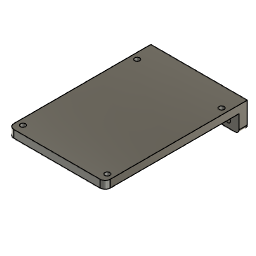
monitor holder v1 (Autodesk Fusion 360 design; units mm, degrees)
Autodesk Fusion 360 part; units mm, degrees
sketch "Sketch1" plane through (0, 0, 0) normal (0, 0, 1) x (1, 0, 0)
  line L0 (0, 0) -> (76, 0)
  line L1 (76, 0) -> (76, 112)
  line L2 (76, 112) -> (0, 112)
  line L3 (0, 112) -> (0, 0)
  circle A0 centre (4.75, 96.5) radius 2
  circle A1 centre (71.25, 96.5) radius 2
  circle A2 centre (71.25, 6.5) radius 2
  circle A3 centre (4.75, 6.5) radius 2
  line L4 (4.75, 96.5) -> (71.25, 96.5) construction
  line L5 (71.25, 96.5) -> (71.25, 6.5) construction
  line L6 (38, 112) -> (38, 0) construction
  dimension "d1" = 76
  dimension "d2" = 112
  dimension "d3" = 66.5
  dimension "d4" = 90
  dimension "d5" = 66.5
  dimension "d6" = 90
  dimension "d7" = 4
  dimension "d8" = 4
  dimension "d9" = 4
  dimension "d10" = 4
  dimension "d11" = 6.5
  constraint horizontal L0
  constraint vertical L1
  constraint horizontal L2
  constraint vertical L3
  constraint coincident L0.start L3.end
  constraint coincident A0.centre L4.start
  constraint coincident A1.centre L4.end
  constraint parallel L2 L4
  constraint coincident A2.centre L5.end
  constraint parallel L1 L5
  constraint midpoint L2 L6.start
  constraint midpoint L0 L6.end
  constraint symmetric A2.centre A3.centre L6
  measures "d1" distance of L0.start L0.end
  measures "d2" distance of L0.end L1.end
  measures "d3" distance of A0.centre A1.centre
  measures "d4" vertical distance of A1.centre A2.centre
  measures "d5" distance of A2.centre A3.centre
  measures "d6" vertical distance of A0.centre A3.centre
  measures "d7" diameter of A0
  measures "d8" diameter of A1
  measures "d9" diameter of A2
  measures "d10" diameter of A3
  measures "d11" distance of L0 A3.centre
extrude "Extrude1" add sketch "Sketch1" along normal blind 6
sketch "Sketch2" plane through (0, 0, 0) normal (0, 0, -1) x (1, 0, 0)
  circle A0 centre (71.25, -96.5) radius 2
  circle A1 centre (4.75, -96.5) radius 2
  circle A2 centre (71.25, -6.5) radius 2
  circle A3 centre (4.75, -6.5) radius 2
  line L0 (0, 0) -> (0, -112)
  line L1 (0, -112) -> (76, -112)
  line L2 (76, -112) -> (76, 0)
  line L3 (76, 0) -> (0, 0)
  line L4 (76, -112) -> (0, -112)
  line L5 (0, -112) -> (0, -105.5)
  line L6 (0, -105.5) -> (76, -105.5)
  line L7 (76, -105.5) -> (76, -112)
  dimension "d14" = 6.5
  constraint horizontal L4
  constraint vertical L5
  constraint horizontal L6
  constraint vertical L7
  constraint coincident L0 L5.end
  constraint coincident L1.end L2.start
  measures "d14" distance of L0.end L5.end
extrude "Extrude2" add sketch "Sketch2" along normal blind 14 contours L0 L1 L2 L4 L5 L6 L7
ref_plane "WorkPlane1" through (53, 56, -4) normal (1, 0, 0) x (0, 1, 0)
sketch "Sketch3" plane through (53, 56, -4) normal (1, 0, 0) x (0, 1, 0)
  line L0 (-56, 4) -> (49.5, 4)
  line L1 (49.5, 4) -> (49.5, -10)
  line L2 (49.5, -10) -> (56, -10)
  line L3 (56, -10) -> (56, 10)
  line L4 (56, 10) -> (-56, 10)
  line L5 (-56, 10) -> (-56, 4)
  line L6 (-56, 4) -> (49.5, 4)
  line L7 (49.5, -10) -> (-27.892, 4)
  constraint coincident L1.end L2.start
  constraint coincident L6 L7.end
extrude "Extrude3" add sketch "Sketch3" along normal mid plane 6 contours L0 L1 L6 L7
ref_plane "WorkPlane2" through (23, 56, -4) normal (-1, 0, 0) x (0, -1, 0)
sketch "Sketch4" plane through (23, 56, -4) normal (-1, 0, 0) x (0, 1, 0)
  line L0 (49.5, -4) -> (49.5, 10)
  line L1 (49.5, 10) -> (-27.892, -4)
  line L2 (-27.892, -4) -> (49.5, -4)
  line L3 (49.5, 10) -> (-27.892, -4)
  constraint coincident L0.end L1.start
  constraint coincident L1.end L2.start
extrude "Extrude4" add sketch "Sketch4" along normal mid plane 6
sketch "Sketch5" plane through (0, 112, 0) normal (0, 1, 0) x (-1, 0, 0)
  line L0 (0, -14) -> (0, 6)
  line L1 (0, 6) -> (-76, 6)
  line L2 (-76, 6) -> (-76, -14)
  line L3 (-76, -14) -> (0, -14)
  circle A0 centre (-67.21, -8.5) radius 2
  line L4 (-38, 6) -> (-38, -14) construction
  circle A1 centre (-8.79, -8.5) radius 2
  dimension "d23" = 4
  dimension "d24" = 4
  dimension "d25" = 58.42
  dimension "d26" = 5.5
  constraint midpoint L1 L4.start
  constraint midpoint L3 L4.end
  constraint symmetric A0 L4 A1
  measures "d23" diameter of A0
  measures "d24" diameter of A1
  measures "d25" distance of A0.centre A1.centre
  measures "d26" distance of L3 A1.centre
extrude "Extrude5" cut sketch "Sketch5" against normal blind 6.5 contours A0 | A1
fillet "Fillet1" radius 4 2 edges at (76, 0, 3) (0, 0, 3)
fillet "Fillet2" radius 3 2 edges at (0, 108.75, -14) (76, 108.75, -14)
